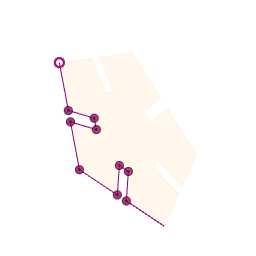
Parametric Construction kit v3 (Autodesk Fusion 360 design; units mm, degrees)
Autodesk Fusion 360 part; units mm, degrees
sketch "Design Sketch" plane through (0, 0, 0) normal (0, 1, 0) x (1, 0, 0)
  circle A0 centre (0, 0) radius 25 construction
  line L0 (0, 0) -> (-23.1195, -9.5125) construction
  line L1 (1.9026, -24.9275) -> (0, 0) construction
  line L2 (1.9026, -24.9275) -> (-23.1195, -9.5125) construction
  line L3 (-10.6084, -17.22) -> (-5.783, -9.3871) construction
  line L4 (-7.1111, -8.5689) -> (-4.4548, -10.2053)
  line L5 (-4.4548, -10.2053) -> (-9.2803, -18.0382)
  line L6 (1.9026, -24.9275) -> (-9.2803, -18.0382)
  line L7 (-7.1111, -8.5689) -> (-11.9366, -16.4018)
  line L8 (-11.9366, -16.4018) -> (-23.1195, -9.5125)
  line L9 (5.952, -9.411) -> (11.9104, -16.4208)
  line L10 (8.3292, -7.3903) -> (14.2876, -14.4002)
  line L11 (5.952, -9.411) -> (8.3292, -7.3903)
  line L12 (11.9104, -16.4208) -> (1.9026, -24.9275)
  line L13 (24.2954, -5.8935) -> (14.2876, -14.4002)
  line L14 (10.7897, 2.7525) -> (19.2977, 6.2531)
  line L15 (9.6025, 5.6378) -> (18.1105, 9.1384)
  line L16 (10.7897, 2.7525) -> (9.6025, 5.6378)
  line L17 (19.2977, 6.2531) -> (24.2954, -5.8935)
  line L18 (13.1128, 21.2851) -> (18.1105, 9.1384)
  line L19 (0.7164, 11.1122) -> (0.0162, 20.2855)
  line L20 (-2.3946, 10.8747) -> (-3.0947, 20.048)
  line L21 (0.7164, 11.1122) -> (-2.3946, 10.8747)
  line L22 (0.0162, 20.2855) -> (13.1128, 21.2851)
  line L23 (-16.1913, 19.0484) -> (-3.0947, 20.048)
  line L24 (-10.3469, 4.1152) -> (-19.2876, 6.284)
  line L25 (-11.0824, 1.0831) -> (-20.0231, 3.2519)
  line L26 (-10.3469, 4.1152) -> (-11.0824, 1.0831)
  line L27 (-19.2876, 6.284) -> (-16.1913, 19.0484)
  line L28 (-23.1195, -9.5125) -> (-20.0231, 3.2519)
  dimension "d1" = 72
  dimension "d4" = 50
  dimension "d5" = 9.2
  dimension "d10" = 360
  dimension "d11" = 3.12
  measures "d1" angle of L0 L1
  measures "d4" diameter of A0
extrude "Extrude1" add sketch "Design Sketch" along normal blind 3.3
sketch "laserCut Output" plane through (0, 0, 0) normal (0, -1, 0) x (1, 0, 0)
  line L0 (-4.4548, 10.2053) -> (-7.1111, 8.5689)
  line L1 (-7.1111, 8.5689) -> (-11.9366, 16.4018)
  line L2 (-11.9366, 16.4018) -> (-23.1195, 9.5125)
  line L3 (13.1128, -21.2851) -> (18.1105, -9.1384)
  line L4 (18.1105, -9.1384) -> (9.6025, -5.6378)
  line L5 (9.6025, -5.6378) -> (10.7897, -2.7525)
  line L6 (10.7897, -2.7525) -> (19.2977, -6.2531)
  line L7 (19.2977, -6.2531) -> (24.2954, 5.8935)
  line L8 (24.2954, 5.8935) -> (14.2876, 14.4002)
  line L9 (14.2876, 14.4002) -> (8.3292, 7.3903)
  line L10 (8.3292, 7.3903) -> (5.952, 9.411)
  line L11 (5.952, 9.411) -> (11.9104, 16.4208)
  line L12 (11.9104, 16.4208) -> (1.9026, 24.9275)
  line L13 (1.9026, 24.9275) -> (-9.2803, 18.0382)
  line L14 (-9.2803, 18.0382) -> (-4.4548, 10.2053)
  line L15 (-16.1913, -19.0484) -> (-3.0947, -20.048)
  line L16 (-3.0947, -20.048) -> (-2.3946, -10.8747)
  line L17 (-2.3946, -10.8747) -> (0.7164, -11.1122)
  line L18 (0.7164, -11.1122) -> (0.0162, -20.2855)
  line L19 (0.0162, -20.2855) -> (13.1128, -21.2851)
  line L20 (-23.1195, 9.5125) -> (-20.0231, -3.2519)
  line L21 (-20.0231, -3.2519) -> (-11.0824, -1.0831)
  line L22 (-11.0824, -1.0831) -> (-10.3469, -4.1152)
  line L23 (-10.3469, -4.1152) -> (-19.2876, -6.284)
  line L24 (-19.2876, -6.284) -> (-16.1913, -19.0484)
hidden bodies 1
equation "d1 = ( 360 / side ) * 1 deg"
equation "side = 5"
equation "length = 50 mm"
equation "d4 = length"
equation "d5 = depth"
equation "depth = ( length / 4 ) - materialThickness"
equation "materialThickness = 3.3 mm"
equation "kerf = ( 0.09 * 2 ) * 1 mm"
equation "d9 = side"
equation "d11 = materialThickness - kerf"
equation "d12 = materialThickness"
